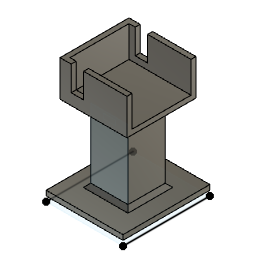
servo support (Autodesk Fusion 360 design; units mm, degrees)
Autodesk Fusion 360 part; units mm, degrees
note: some values were not read from the file. Chosen so that the rebuilt part matches the saved one: which face or edge a step refers to.
sketch "Sketch1" plane through (0, 0, 0) normal (0, 0, 1) x (1, 0, 0)
  line L0 (0, 0) -> (27, 0)
  line L1 (27, 0) -> (27, 27.8)
  line L2 (27, 27.8) -> (0, 27.8)
  line L3 (0, 27.8) -> (0, 0)
  dimension "d1" = 27.8
  dimension "d2" = 27
  constraint horizontal L0
  constraint vertical L1
  constraint horizontal L2
  constraint vertical L3
  constraint coincident L0.start L3.end
  measures "d1" distance of L0.start L2.end
  measures "d2" distance of L0.start L0.end
sketch "Sketch2" plane through (0, 0, 0) normal (0, 0, 1) x (1, 0, 0)
extrude "Extrude1" add sketch "Sketch1" along normal blind 14.5
shell "Shell1" thickness 2 removed faces 1 at (9, 18.5333, 14.5)
sketch "Sketch3" plane through (27, 0, 0) normal (1, 0, 0) x (0, 1, 0)
  line L0 (0, 0) -> (27.8, 0)
  line L1 (27.8, 0) -> (27.8, 14.5)
  line L2 (27.8, 14.5) -> (0, 14.5)
  line L3 (0, 14.5) -> (0, 0)
  line L4 (2, 14.5) -> (25.8, 14.5)
  line L5 (25.8, 14.5) -> (25.8, 2)
  line L6 (25.8, 2) -> (2, 2)
  line L7 (2, 2) -> (2, 14.5)
  dimension "d6" = 23.8
  dimension "d7" = 2
  dimension "d8" = 2
  constraint horizontal L4
  constraint vertical L5
  constraint horizontal L6
  constraint vertical L7
  constraint coincident L2 L4.start
  measures "d6" distance of L4.start L4.end
  measures "d7" distance of L3 L7
  measures "d8" distance of L0 L6
extrude "Extrude2" cut sketch "Sketch3" against normal blind 2 contours L2 L4 L5 L6 L7
sketch "Sketch4" plane through (0, 0, 0) normal (0, -1, 0) x (1, 0, 0)
  line L0 (0, 0) -> (27, 0)
  line L1 (27, 0) -> (27, 14.5)
  line L2 (27, 14.5) -> (0, 14.5)
  line L3 (0, 14.5) -> (0, 0)
  line L4 (4.5, 14.5) -> (9.5, 14.5)
  line L5 (9.5, 14.5) -> (9.5, 4.5)
  line L6 (9.5, 4.5) -> (4.5, 4.5)
  line L7 (4.5, 4.5) -> (4.5, 14.5)
  dimension "d11" = 4.5
  dimension "d12" = 5
  dimension "d13" = 10
  constraint horizontal L4
  constraint vertical L5
  constraint horizontal L6
  constraint vertical L7
  constraint coincident L2 L4.start
  measures "d11" distance of L3 L7
  measures "d12" distance of L5 L7
  measures "d13" distance of L4 L6
extrude "Extrude3" cut sketch "Sketch4" against normal blind 40 contours L2 L4 L5 L6 L7
sketch "Sketch5" plane through (0, 0, 0) normal (0, 0, -1) x (1, 0, 0)
  line L0 (0, 0) -> (0, -27.8)
  line L1 (0, -27.8) -> (27, -27.8)
  line L2 (27, -27.8) -> (27, 0)
  line L3 (27, 0) -> (0, 0)
  line L4 (6, -6.4) -> (21, -6.4)
  line L5 (21, -6.4) -> (21, -21.4)
  line L6 (21, -21.4) -> (6, -21.4)
  line L7 (6, -21.4) -> (6, -6.4)
  dimension "d16" = 6
  dimension "d17" = 15
  dimension "d18" = 15
  dimension "d19" = 6.4
  constraint horizontal L4
  constraint vertical L5
  constraint horizontal L6
  constraint vertical L7
  measures "d16" distance of L0 L7
  measures "d17" distance of L5 L7
  measures "d18" distance of L4 L6
  measures "d19" distance of L1 L6
extrude "Extrude4" add sketch "Sketch5" along normal blind 35 contours L4 L5 L6 L7
sketch "Sketch6" plane through (0, 0, -35) normal (0, 0, -1) x (1, 0, 0)
  line L0 (6, -21.4) -> (21, -21.4)
  line L1 (21, -21.4) -> (21, -6.4)
  line L2 (21, -6.4) -> (6, -6.4)
  line L3 (6, -6.4) -> (6, -21.4)
  line L4 (9, -9.4) -> (18, -9.4)
  line L5 (18, -9.4) -> (18, -18.4)
  line L6 (18, -18.4) -> (9, -18.4)
  line L7 (9, -18.4) -> (9, -9.4)
  dimension "d29" = 3
  dimension "d30" = 3
  dimension "d31" = 3
  dimension "d32" = 3
  constraint horizontal L4
  constraint vertical L5
  constraint horizontal L6
  constraint vertical L7
  measures "d29" distance of L2 L4
  measures "d30" distance of L3 L7
  measures "d31" distance of L0 L6
  measures "d32" distance of L1 L5
extrude "Extrude5" add sketch "Sketch6" against normal blind 2
chamfer "Chamfer1" distance 1.5 angle 45 4 edges at (6, 13.9, 0) (13.5, 6.4, 0) (13.5, 21.4, 0) (21, 13.9, 0)
extrude "Extrude6" cut sketch "Sketch6" against normal blind 33 contours L4 L5 L6 L7
sketch "Sketch8" plane through (0, 0, -35) normal (0, 0, -1) x (1, 0, 0)
  line L0 (-2, 3.6) -> (29, 3.6)
  line L1 (29, 3.6) -> (29, -31.4)
  line L2 (29, -31.4) -> (-2, -31.4)
  line L3 (-2, -31.4) -> (-2, 3.6)
  line L4 (9, -18.4) -> (9, -9.4)
  line L5 (9, -9.4) -> (18, -9.4)
  line L6 (6, -21.4) -> (21, -21.4)
  line L7 (18, -9.4) -> (18, -18.4)
  line L8 (18, -18.4) -> (9, -18.4)
  dimension "d39" = 11
  dimension "d40" = 13
  dimension "d42" = 11
  dimension "d43" = 13
  constraint horizontal L0
  constraint vertical L1
  constraint horizontal L2
  constraint vertical L3
  measures "d39" distance of L3 L4
  measures "d40" distance of L0 L5
  measures "d42" distance of L1 L7
  measures "d43" distance of L2 L8
extrude "Extrude7" add sketch "Sketch8" against normal blind 2 contours L0 L1 L2 L3 | L4 L5 L7 L8
chamfer "Chamfer2" distance 1.5 angle 45 4 edges at (21, 13.9, -33) (13.5, 6.4, -33) (13.5, 21.4, -33) (6, 13.9, -33)
sketch "Sketch9" plane through (0, 6.4, 0) normal (0, -1, 0) x (1, 0, 0)
  line L0 (6, -31.5) -> (21, -31.5)
  line L1 (21, -31.5) -> (21, -1.5)
  line L2 (21, -1.5) -> (6, -1.5)
  line L3 (6, -1.5) -> (6, -31.5)
  line L4 (11, -2.5) -> (16, -2.5)
  line L5 (16, -2.5) -> (16, -4.5)
  line L6 (16, -4.5) -> (11, -4.5)
  line L7 (11, -4.5) -> (11, -2.5)
  dimension "d47" = 1
  dimension "d48" = 2
  dimension "d49" = 5
  dimension "d50" = 5
  constraint horizontal L4
  constraint vertical L5
  constraint horizontal L6
  constraint vertical L7
  measures "d47" distance of L2 L4
  measures "d48" distance of L4 L6
  measures "d49" distance of L5 L7
  measures "d50" distance of L3 L7
extrude "Extrude8" cut sketch "Sketch9" against normal blind 30 contours L4 L5 L6 L7
sketch "Sketch10" plane through (0, 6.4, 0) normal (0, -1, 0) x (1, 0, 0)
  line L0 (16, -2.5) -> (16, -4.5)
  line L1 (16, -4.5) -> (11, -4.5)
  line L2 (11, -4.5) -> (11, -2.5)
  line L3 (11, -2.5) -> (16, -2.5)
  line L4 (6, -31.5) -> (21, -31.5)
  line L5 (21, -31.5) -> (21, -1.5)
  line L6 (21, -1.5) -> (6, -1.5)
  line L7 (6, -1.5) -> (6, -31.5)
sketch "Sketch11" plane through (0, 0, -35) normal (0, 0, -1) x (1, 0, 0)
  line L0 (-2, -31.4) -> (29, -31.4)
  line L1 (29, -31.4) -> (29, 3.6)
  line L2 (29, 3.6) -> (-2, 3.6)
  line L3 (-2, 3.6) -> (-2, -31.4)
  line L4 (-2, -31.4) -> (-2, 3.6)
  line L5 (29, 3.6) -> (29, -31.4)
  constraint coincident L0.start L3.end
  constraint coincident L2.end L3.start
  constraint coincident L1.end L2.start
  constraint coincident L0.end L1.start
extrude "Extrude9" add sketch "Sketch11" against normal blind 4
extrude "Extrude10" cut sketch "Sketch11" against normal blind 2
chamfer "Chamfer3" distance 1.5 angle 45 4 edges at (13.5, 6.4, -31) (21, 13.9, -31) (13.5, 21.4, -31) (6, 13.9, -31)
sketch "Sketch12" plane through (0, 6.4, 0) normal (0, -1, 0) x (1, 0, 0)
